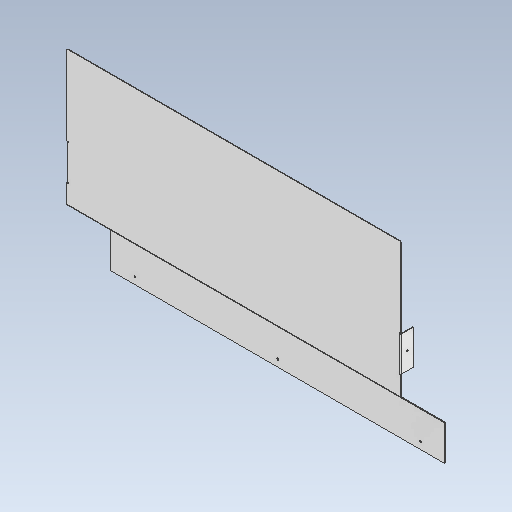
# Autodesk Inventor part: Tapa_blanca_trasera
Saved by Autodesk Inventor 2021 (Build 250183000, 183)
## iProperties
Created: 2021-04-16
Part Number: Tapa_blanca_trasera
Material: Acero AISI 1006 85 LC
Document SubType Name: Chapa
Designer: Admin
Density: 7.872 g/cm^3
Sheet Metal Rule: Por defecto_mm
Appearance: Blanco
Mass: 1402.87 g
Surface Area: 3934.28 cm^2
Volume: 178.21 cm^3
Author: Admin
Autodesk Inventor part; units mm, degrees
ref_plane "YZ Plane" through (0, 0, 0) normal (1, 0, 0) x (0, 1, 0)
ref_plane "XZ Plane" through (0, 0, 0) normal (0, 1, 0) x (-1, 0, 0)
ref_plane "XY Plane" through (0, 0, 0) normal (0, 0, 1) x (1, 0, 0)
sketch "Boceto1" plane through (0, 0, 0) normal (0, 0, 1) x (1, 0, 0)
  line L0 (0, 0) -> (527.58, 0)
  line L1 (0, 0) -> (0, 56.2)
  line L2 (527.58, 0) -> (527.58, 56.2)
  line L3 (527.58, 56.2) -> (0, 56.2)
  dimension "d0" = 527.58
  dimension "d1" = 56.2
  dimension "d2" = 56.2
  measures "d0" distance of L0.start L0.end
  measures "d1" distance of L0.start L1.end
  measures "d2" distance of L0.end L2.end
extrude "Placa1" add sketch "Boceto1" along normal blind 0.91
sketch "Boceto2" plane through (0, 55.5556, 0.6426) normal (0, 0.7080934, -0.7061188) x (-1, 0, 0)
  line L0 (-527.58, 0) -> (0, 0)
  line L1 (0, 0) -> (0, 98.854)
  line L2 (0, 98.854) -> (-527.58, 98.854)
  line L3 (-527.58, 98.854) -> (-527.58, 0)
  constraints: 6 end point, 1 horizontal, 1 perpendicular, 1 vertical
edge flange "Pestaña1" height 98.854 angle 45.08 thickness 0.91 bend radius 0.91 thickness toward (0, 0.7080934, -0.7061188) relief straight relief width 0.91 relief depth 0.455 edges at (263.79, 56.2, 0.91) wall of the first edge with corners at (527.58, 55.5556, 0.6426) (0, 55.5556, 0.6426) (0, 125.3583, 70.6404) (527.58, 125.3583, 70.6404)
bend "Doblez1"
corner "Esquina1"
sketch "Boceto3" plane through (0, 125.3583, 69.7304) normal (0, 0, 1) x (-1, 0, 0)
  line L0 (-527.58, 0) -> (0, 0)
  line L1 (0, 0) -> (0, 213.25)
  line L2 (0, 213.25) -> (-527.58, 213.25)
  line L3 (-527.58, 213.25) -> (-527.58, 0)
  constraints: 6 end point, 1 horizontal, 1 perpendicular, 1 vertical
edge flange "Pestaña2" height 213.25 angle -45.08 thickness 0.91 bend radius 0.91 thickness toward (0, 0, 1) relief straight relief width 0.91 relief depth 0.455 edges at (263.79, 125.3583, 70.6404) wall of the first edge with corners at (527.58, 125.3583, 69.7304) (0, 125.3583, 69.7304) (0, 338.6083, 69.7304) (527.58, 338.6083, 69.7304)
bend "Doblez2"
corner "Esquina2"
sketch "Boceto4" plane through (0, 126.1137, 70.6404) normal (-1, 0, 0) x (0, 0, 1)
  line L0 (0, 0) -> (0, 212.4946)
  line L1 (0, 85.3289) -> (-20, 85.3289)
  line L2 (-20, 85.3289) -> (-20, 30.3289)
  line L3 (-20, 30.3289) -> (0, 30.3289)
  line L4 (0, 30.3289) -> (0, 85.3289)
  point P0 (-70.6404, -126.1137)
  dimension "d24" = 20
  dimension "d25" = 55
  measures "d24" distance of L3.end L2.end
  measures "d25" distance of L2.end L1.end
sheet face with bend "Cara2" sketch "Boceto4" thickness 0.91 toward (1, 0, 0) bend radius 0.91 relief straight relief width 0.91 relief depth 0.455
bend "Doblez3"
sketch "Boceto5" plane through (527.58, 126.1137, 69.7304) normal (1, 0, 0) x (0, 0, -1)
  line L0 (-0.91, 85.3289) -> (0, 85.3289)
  line L1 (19.09, 85.3289) -> (19.09, 30.3289)
  line L2 (-0.91, 85.3289) -> (19.09, 85.3289)
  line L3 (19.09, 85.3289) -> (19.09, 30.3289)
  line L4 (19.09, 30.3289) -> (-0.91, 30.3289)
  line L5 (-0.91, 30.3289) -> (-0.91, 85.3289)
  point P0 (69.7304, -126.1137)
sheet face with bend "Cara3" sketch "Boceto5" thickness 0.91 toward (-1, 0, 0) bend radius 0.91 relief straight relief width 0.91 relief depth 0.455
bend "Doblez4"
fillet "Redondeo de esquina1" radius 1.5 1 edges at (527.58, 338.6083, 70.1854)
fillet "Redondeo de esquina2" radius 1.5 1 edges at (0, 338.6083, 70.1854)
sketch "Boceto6" plane through (527.58, 126.1137, 69.7304) normal (1, 0, 0) x (0, 0, -1)
  line L0 (19.09, 85.3289) -> (19.09, 30.3289) construction
  line L1 (0, 86.2389) -> (0, 85.3289) construction
  line L2 (19.09, 30.3289) -> (0, 85.3289) construction
  line L3 (0, 30.3289) -> (0, 29.4189) construction
  line L4 (0, 30.3289) -> (19.09, 85.3289) construction
  circle A0 centre (9.545, 57.8289) radius 1.5875
  point P0 (69.7304, -126.1137)
  dimension "d38" = 3.175
  constraints: 4 end point, 1 centre point, 1 midpoint
  measures "d38" diameter of A0
extrude "Cortar1" cut sketch "Boceto6" against normal blind 0.91
sketch "Boceto7" plane through (0, 126.1137, 70.6404) normal (-1, 0, 0) x (0, 0, 1)
  line L0 (-1.82, 30.3289) -> (-20, 30.3289) construction
  line L1 (-20, 85.3289) -> (-1.82, 30.3289) construction
  line L2 (-1.82, 85.3289) -> (-0.91, 85.3289) construction
  line L3 (-20, 30.3289) -> (-1.82, 85.3289) construction
  circle A0 centre (-10.91, 57.8289) radius 1.5875
  point P0 (-70.6404, -126.1137)
  dimension "d41" = 3.175
  constraints: 4 end point, 1 centre point, 1 midpoint
  measures "d41" diameter of A0
extrude "Cortar2" cut sketch "Boceto7" against normal blind 0.91
sketch "Boceto8" plane through (0, 0, 0.91) normal (0, 0, 1) x (1, 0, 0)
  circle A0 centre (489.48, 10.8421) radius 1.5875 projected
  circle A1 centre (263.79, 10.8421) radius 1.5875 projected
  circle A2 centre (38.1, 10.8421) radius 1.5875 projected
  point P0 (0, 0)
extrude "Cortar3" cut sketch "Boceto8" against normal blind 0.91
equation "\"d39\" = Grosor"
equation "\"d42\" = Grosor"
equation "\"d44\" = Grosor"
equation "\"d3\" = Grosor"
equation "\"d4\" = Anchura_desahogo_plegado"
equation "\"d5\" = Profundidad_desahogo_plegado"
equation "\"d6\" = Remanente_mínimo"
equation "\"d7\" = Radiodetransición"
equation "\"d10\" = Radio_pliegue"
equation "\"d11\" = Tamaño_destalonado"
equation "\"d12\" = TamañoSeparación"
equation "\"d13\" = Tamaño_de_radio_de_Jacobi"
equation "\"d14\" = Anchura_desahogo_plegado"
equation "\"d15\" = Profundidad_desahogo_plegado"
equation "\"d16\" = Remanente_mínimo"
equation "\"d17\" = Radiodetransición"
equation "\"d20\" = Radio_pliegue"
equation "\"d21\" = Tamaño_destalonado"
equation "\"d22\" = TamañoSeparación"
equation "\"d23\" = Tamaño_de_radio_de_Jacobi"
equation "\"d26\" = Radio_pliegue"
equation "\"d27\" = Anchura_desahogo_plegado"
equation "\"d29\" = Remanente_mínimo"
equation "\"d28\" = Profundidad_desahogo_plegado"
equation "\"d30\" = Radiodetransición"
equation "\"d31\" = Radio_pliegue"
equation "\"d32\" = Anchura_desahogo_plegado"
equation "\"d34\" = Remanente_mínimo"
equation "\"d33\" = Profundidad_desahogo_plegado"
equation "\"d35\" = Radiodetransición"
equation "\"Radio_pliegue\" = Grosor"
equation "\"Anchura_desahogo_plegado\" = Grosor"
equation "\"Profundidad_desahogo_plegado\" = 0.5 * Grosor"
equation "\"Tamaño_destalonado\" = 4 * Grosor"
equation "\"Remanente_mínimo\" = 2 * Grosor"
equation "\"Radiodetransición\" = Radio_pliegue"
equation "\"Tamaño_de_radio_de_Jacobi\" = Radio_pliegue"
equation "\"TamañoSeparación\" = Grosor"
equation "\"Grosor\" = 0.91"
